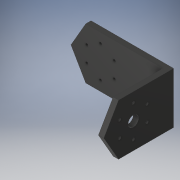
# Autodesk Inventor part: TARM03
Saved by Autodesk Inventor 2017 (Build 210142000, 142)
## iProperties
Created: 2018-10-19
Part Number: TARM03
Material: ABS Plastic
Document SubType Name: Modeling
Designer: Dell
Density: 1.06 g/cm^3
Appearance: Smooth - Black
Author: Dell
Autodesk Inventor part; units mm, degrees
ref_plane "YZ Plane" through (0, 0, 0) normal (1, 0, 0) x (0, 1, 0)
ref_plane "XZ Plane" through (0, 0, 0) normal (0, 1, 0) x (-1, 0, 0)
ref_plane "XY Plane" through (0, 0, 0) normal (0, 0, 1) x (1, 0, 0)
sketch "Sketch1" plane through (0, 0, 0) normal (0, 0, 1) x (1, 0, 0)
  line L0 (-56, 0) -> (-28, 48.4974)
  line L1 (-28, 48.4974) -> (28, 48.4974)
  line L2 (28, 48.4974) -> (56, 0)
  line L3 (56, 0) -> (28, -48.4974)
  line L4 (28, -48.4974) -> (-28, -48.4974)
  line L5 (-28, -48.4974) -> (-56, 0)
  circle A0 centre (0, 30) radius 2.5
  circle A1 centre (-25.9808, 15) radius 2.5
  circle A2 centre (-25.9808, -15) radius 2.5
  circle A3 centre (0, -30) radius 2.5
  circle A4 centre (25.9808, -15) radius 2.5
  circle A5 centre (25.9808, 15) radius 2.5
  point P0 (0, 0)
  point P1 (0, 0)
  dimension "d0" = 112
  dimension "d1" = 5
  dimension "d2" = 30
  dimension "d5" = 360
  constraints: 12 end point, 6 centre point, 1 coincident, 1 horizontal alignment, 1 vertical alignment, 26 other
  measures "d0" distance of L2.end L0.start
  measures "d1" diameter of A0
  measures "d2" distance of point (0, 0) A0.centre
extrude "Extrusion1" add sketch "Sketch1" along normal blind 10
sketch "Sketch2" plane through (0, 0, 10) normal (0, 0, 1) x (1, 0, 0)
  line L0 (28, 48.4974) -> (-28, 48.4974) projected
  line L1 (28, 48.4974) -> (128, 48.4974)
  line L2 (128, 48.4974) -> (128, -48.4974)
  line L3 (128, -48.4974) -> (28, -48.4974)
  circle A0 centre (25.9808, 15) radius 2.5 projected
  circle A1 centre (25.9808, -15) radius 2.5 projected
  line L4 (56, 0) -> (28, 48.4974) projected
  line L5 (28, -48.4974) -> (56, 0) projected
  line L6 (-28, -48.4974) -> (28, -48.4974) projected
  line L7 (28, -48.4974) -> (56, 0)
  line L8 (28, 48.4974) -> (56, 0)
  line L9 (28, -48.4974) -> (128, -48.4974)
  line L10 (28, 48.4974) -> (128, 48.4974)
  point P0 (0, 0)
  dimension "d10" = 100
  constraints: 14 end point, 3 equal length, 1 horizontal, 1 horizontal alignment, 1 perpendicular
  measures "d10" distance from line of L2 L0.start
extrude "Extrusion2" add sketch "Sketch2" against normal blind 10 contours L1 L2 L3 L5 L4
sketch "Sketch3" plane through (128, -48.4974, 10) normal (1, 0, 0) x (0, 0, -1)
  line L0 (0, 0) -> (0, 96.9948) projected
  line L1 (-38, 96.9948) -> (-10, 48.4974)
  line L2 (-10, 48.4974) -> (-38, 0)
  line L3 (-38, 0) -> (-94, 0)
  line L4 (-94, 0) -> (-122, 48.4974)
  line L5 (-122, 48.4974) -> (-94, 96.9948)
  line L6 (-94, 96.9948) -> (-38, 96.9948)
  line L7 (0, 0) -> (-38, 0)
  line L8 (-38, 0) -> (-38, 96.9948) construction
  line L9 (-38, 96.9948) -> (0, 96.9948)
  line L10 (0, 96.9948) -> (0, 0)
  circle A0 centre (-66, 78.4974) radius 2.5
  circle A1 centre (-91.9808, 63.4974) radius 2.5
  circle A2 centre (-91.9808, 33.4974) radius 2.5
  circle A3 centre (-66, 18.4974) radius 2.5
  circle A4 centre (-40.0192, 33.4974) radius 2.5
  circle A5 centre (-40.0192, 63.4974) radius 2.5
  line L11 (-38, 0) -> (-10, 48.4974)
  line L12 (-10, 48.4974) -> (-38, 96.9948)
  line L13 (-38, 96.9948) -> (0, 96.9948)
  line L14 (0, 48.4974) -> (0, 0) projected
  line L15 (-38, 0) -> (0, 0)
  circle A6 centre (-66, 48.4974) radius 10
  point P0 (10, 48.4974)
  dimension "d17" = 112
  dimension "d18" = 10
  dimension "d19" = 5
  dimension "d20" = 30
  dimension "d23" = 360
  dimension "d27" = 20
  constraints: 28 end point, 7 centre point, 4 equal length, 3 horizontal, 1 coincident, 1 perpendicular, 1 vertical alignment, 26 other
  measures "d17" distance of L1.end L4.end
  measures "d18" distance from line of L0 L1.end
  measures "d19" diameter of A0
  measures "d20" distance of A0.centre point (-66, 48.497)
  measures "d27" diameter of A6
extrude "Extrusion3" add sketch "Sketch3" against normal blind 10
body "Solid1"
